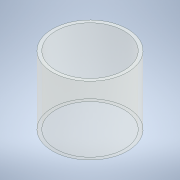
# Autodesk Inventor part: tube001_beta
Saved by Autodesk Inventor 2020 (Build 240168000, 168)
## iProperties
Created: 2024-01-17
Part Number: tube001_beta
Material: Стекло
Document SubType Name: Modeling
Designer: 4s
Density: 2.18 g/cm^3
Appearance: Бесцветный
Author: 4s
Autodesk Inventor part; units mm, degrees
ref_plane "YZ Plane" through (0, 0, 0) normal (1, 0, 0) x (0, 1, 0)
ref_plane "XZ Plane" through (0, 0, 0) normal (0, 1, 0) x (-1, 0, 0)
ref_plane "XY Plane" through (0, 0, 0) normal (0, 0, 1) x (1, 0, 0)
sketch "Эскиз1" plane through (0, 0, 0) normal (0, 1, 0) x (-1, 0, 0)
  circle A0 centre (0, 0) radius 20
  circle A1 centre (0, 0) radius 22
  dimension "d0" = 40
  dimension "d1" = 2
  constraints: 2 centre point, 2 coincident
  measures "d0" diameter of A0
  measures "d1" radial gap between concentric circles of A1 A0
extrude "Выдавливание1" add sketch "Эскиз1" along normal blind 40
